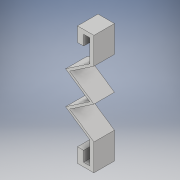
# Autodesk Inventor part: Spring Mk 1
Saved by Autodesk Inventor 2019 (Build 230136000, 136)
## iProperties
Created: 2019-02-23
Part Number: Spring Mk 1
Material: Generic
Document SubType Name: Modeling
Designer: Kepler
Density: 1 g/cm^3
Appearance: Default
Author: Kepler
Autodesk Inventor part; units mm, degrees
ref_plane "YZ Plane" through (0, 0, 0) normal (1, 0, 0) x (0, 1, 0)
ref_plane "XZ Plane" through (0, 0, 0) normal (0, 1, 0) x (-1, 0, 0)
ref_plane "XY Plane" through (0, 0, 0) normal (0, 0, 1) x (1, 0, 0)
sketch "Sketch1" plane through (0, 0, 0) normal (0, 0, 1) x (1, 0, 0)
  line L0 (0, 0) -> (0, 3.5)
  line L1 (0, 3.5) -> (1.5, 3.5)
  line L2 (1.5, 3.5) -> (1.5, 1)
  line L3 (1.5, 1) -> (3, 1)
  line L4 (3, 1) -> (3, 6.5)
  line L5 (0, 0) -> (4, 0)
  line L6 (4, 0) -> (4, 6.5)
  line L7 (3, 6.5) -> (-2.9089, 10.5)
  line L8 (4, 6.5) -> (-1.9089, 10.5)
  line L9 (-2.9089, 10.5) -> (3, 14.5)
  line L10 (-1.9089, 10.5) -> (4, 14.5)
  line L11 (4.8688, 14.5) -> (7.9989, 14.5)
  line L12 (2, 10.5) -> (4.7625, 10.5)
  line L13 (0, 29) -> (0, 25.5)
  line L14 (0, 25.5) -> (1.5, 25.5)
  line L15 (1.5, 25.5) -> (1.5, 28)
  line L16 (1.5, 28) -> (3, 28)
  line L17 (3, 28) -> (3, 22.5)
  line L18 (0, 29) -> (4, 29)
  line L19 (4, 29) -> (4, 22.5)
  line L20 (3, 22.5) -> (-2.9089, 18.5)
  line L21 (4, 22.5) -> (-1.9089, 18.5)
  line L22 (-2.9089, 18.5) -> (3, 14.5)
  line L23 (-1.9089, 18.5) -> (4, 14.5)
  line L24 (2, 18.5) -> (4.7625, 18.5)
  dimension "d0" = 3.5
  dimension "d1" = 1.5
  dimension "d2" = 2.5
  dimension "d3" = 1.5
  dimension "d4" = 5.5
  dimension "d5" = 4
  dimension "d7" = 6.5
  dimension "d8" = 0
  dimension "d10" = 8
  dimension "d11" = 4
  constraints: 50 end point, 13 symmetric about line, 4 vertical, 3 parallel, 3 perpendicular, 2 horizontal, 1 other
  measures "d0" distance of L0.start L0.end
  measures "d1" distance of L0.end L1.end
  measures "d2" distance of L1.end L2.end
  measures "d3" distance of L2.end L3.end
  measures "d4" distance of L3.end L4.end
  measures "d5" distance of L0.start L5.end
  measures "d7" distance of L5.end L6.end
  measures "d8" distance from line of L10.end L6
  measures "d10" distance from line of L11 L6.end
  measures "d11" distance from line of L6.end L12
extrude "Extrusion1" add sketch "Sketch1" along normal blind 5
equation "\"d10\" = 2 * d11"
body "Solid1"
